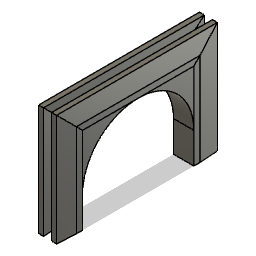
cover-edges-stepper-arch (Autodesk Fusion 360 design; units mm, degrees)
Autodesk Fusion 360 part; units mm, degrees
sketch "Sketch1" plane through (0, 0, 0) normal (0, 0, 1) x (1, 0, 0)
  line L0 (0, 7.5) -> (0, -2.5) construction
  line L1 (-4.125, 0) -> (4.125, 0) construction
  line L2 (-3.625, 7.5) -> (-4.125, 0)
  line L3 (-4.125, -2.5) -> (4.125, -2.5)
  line L4 (4.125, -2.5) -> (4.125, 0)
  line L5 (4.125, 0) -> (3.625, 7.5)
  line L6 (3.625, 7.5) -> (1.625, 7.5)
  line L7 (1.625, 7.5) -> (2.125, 0)
  line L8 (-2.125, 0) -> (-1.625, 7.5)
  line L9 (-1.625, 7.5) -> (-3.625, 7.5)
  line L10 (-2.125, 0) -> (2.125, 0)
  line L11 (-3.8098, 4.7284) -> (-1.8142, 4.5954) construction
  line L12 (-4.125, 0) -> (-4.125, -2.5)
  dimension "d7" = 7.5
  dimension "d8" = 8.25
  dimension "d9" = 4.25
  dimension "d10" = 3.25
  dimension "d12" = 2
  dimension "d13" = 2.5
  constraint vertical L0
  constraint perpendicular L0 L1
  constraint horizontal origin L1.end
  constraint vertical origin L0.start
  constraint symmetric L0 L1.start L1.end
  constraint perpendicular L4 L6
  constraint coincident L1 L7.end
  constraint coincident L1 L8.start
  constraint symmetric L0 L7.end L8.start
  constraint horizontal L9
  constraint horizontal L6
  constraint horizontal L6.end L8.end
  constraint symmetric L0 L6.end L8.end
  constraint horizontal L0.start L8.end
  constraint parallel L2 L8
  constraint parallel L5 L7
  constraint coincident L2 L11.start
  constraint perpendicular L8 L11
  constraint perpendicular L1 L12
  constraint horizontal L3
  constraint coincident L3.end L4.start
  constraint coincident L3 L0.end
  measures "d7" distance of origin L0.start
  measures "d8" distance of L1.start L1.end
  measures "d9" distance of L7.end L8.start
  measures "d10" distance of L6.end L8.end
  measures "d12" distance of L11.start L11.end
  measures "d13" distance of origin L0.end
extrude "Extrude1" add sketch "Sketch1" along normal blind 65 makes body 1
ref_plane "WorkPlane1" through (0, -2.5, 0) normal (0, -0.707107, 0.707107) x (1, 0, 0)
ref_plane "WorkPlane4" through (-2.625, 7.5, 0) normal (0, 0.707107, 0.707107) x (-1, 0, 0)
sketch "Sketch4" plane through (-2.625, 7.5, 0) normal (0, 0.707107, 0.707107) x (-1, 0, 0)
  line L0 (-13, -5) -> (9, -5)
  line L1 (9, -5) -> (9, 21.8685)
  line L2 (9, 21.8685) -> (-13, 21.8685)
  line L3 (-13, 21.8685) -> (-13, -5)
  constraint horizontal L0
  constraint vertical L1
  constraint horizontal L2
  constraint vertical L3
extrude "Extrude5" cut sketch "Sketch4" against normal through all bodies 1
ref_plane "WorkPlane5" through (2.625, 7.5, 65) normal (0, -0.707107, 0.707107) x (-1, 0, 0)
sketch "Sketch5" plane through (2.625, -2.5, 55) normal (0, -0.707107, 0.707107) x (-1, 0, 0)
  line L0 (11.3254, -19.5317) -> (-9, -19.5317)
  line L1 (-9, -19.5317) -> (-9, 23.4955)
  line L2 (-9, 23.4955) -> (11.3254, 23.4955)
  line L3 (11.3254, 23.4955) -> (11.3254, -19.5317)
  constraint horizontal L0
  constraint vertical L1
  constraint horizontal L2
  constraint vertical L3
extrude "Extrude6" cut sketch "Sketch5" along normal through all bodies 1
extrude "Extrude7" add sketch "Sketch1" against normal blind 45 separate body makes body 2
move_body "Move3" bodies 2 to x (1, 0, 0) y (0, 0, -1) z (0, 1, 0) at (0, 7.5, 7.5)
sketch "Sketch7" plane through (-2.625, 7.5, 0) normal (0, 0.707107, 0.707107) x (-1, 0, 0)
  line L0 (-8.5, -5) -> (4.5717, -5)
  line L1 (4.5717, -5) -> (4.5717, 17.417)
  line L2 (4.5717, 17.417) -> (-8.5, 17.417)
  line L3 (-8.5, 17.417) -> (-8.5, -5)
  constraint horizontal L0
  constraint vertical L1
  constraint horizontal L2
  constraint vertical L3
extrude "Extrude9" cut sketch "Sketch7" along normal through all bodies 2
extrude "Extrude10" add sketch "Sketch1" along normal blind 45 separate body makes body 3
move_body "Move4" bodies 3 to x (1, 0, 0) y (0, 0, 1) z (0, -1, 0) at (0, 7.5, 57.5)
sketch "Sketch8" plane through (2.625, 7.5, 65) normal (0, -0.707107, 0.707107) x (-1, 0, 0)
  line L0 (24, -12) -> (-21, -12)
  line L1 (-21, -12) -> (-21, 27)
  line L2 (-21, 27) -> (24, 27)
  line L3 (24, 27) -> (24, -12)
  constraint horizontal L0
  constraint vertical L1
  constraint horizontal L2
  constraint vertical L3
extrude "Extrude11" cut sketch "Sketch8" against normal through all bodies 3
sketch "Sketch9" plane through (-4.125, 0, 0) normal (-1, 0, 0) x (0, 0, 1)
  line L0 (55, -2.5) -> (57.5, 0)
  line L1 (57.5, 0) -> (7.5, 0)
  line L2 (7.5, 0) -> (10, -2.5)
  line L3 (10, -2.5) -> (55, -2.5)
  circle A0 centre (32.5, -25) radius 22.5
  circle A1 centre (32.5, -25) radius 22.5
  line L4 (10, -25) -> (10, -7.1601)
  line L5 (10, -7.1601) -> (10, -2.5)
  line L6 (10, -2.5) -> (32.5, -2.5)
  line L7 (32.5, -2.5) -> (55, -2.5)
  line L8 (55, -2.5) -> (55, -25)
  constraint horizontal A0.centre A1.centre
  constraint equal A0 A1
  constraint vertical L4
  constraint perpendicular L3 L5
  constraint perpendicular L5 L6
  constraint tangent A0 L6
  constraint tangent A0 L5
  constraint horizontal A0.centre L4.start
  constraint vertical A0.centre L6.end
  constraint horizontal L7
  constraint coincident A1 L6.end
  constraint coincident A1 L8.end
  constraint horizontal A0.centre L8.end
  constraint tangent A1 L8
  constraint coincident L2.end L3.start
  constraint coincident L0.start L3.end
  constraint coincident A0.centre A1.centre
extrude "Extrude12" add sketch "Sketch9" against normal blind 8.25 separate body contours L3 A0 A1 L7 L8 | L3 A0 A1 L4 L5 L6 makes body 4 at (1.375, -23.9294, 10.0255)
equation "thickness_back = 2.5 mm"
equation "thickness_sides = 2 mm"
equation "length_sides = 7.5 mm"
equation "width_normal = 4.25 mm"
equation "width_pinch = 3.25 mm"
equation "d7 = length_sides"
equation "d8 = width_normal + 2 * thickness_sides"
equation "d9 = width_normal"
equation "d10 = width_pinch"
equation "d12 = thickness_sides"
equation "d13 = thickness_back"
equation "d35 = -width_normal - 2 * thickness_sides"
